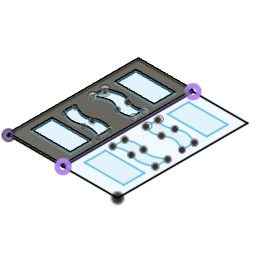
flaps final v2 (Autodesk Fusion 360 design; units mm, degrees)
Autodesk Fusion 360 part; units mm, degrees
sketch "Sketch1" plane through (0, 0, 0) normal (0, 0, 1) x (1, 0, 0)
  line L0 (0, 500) -> (0, 0)
  line L1 (0, 0) -> (210, 0)
  line L2 (210, 0) -> (210, 500)
  line L3 (210, 500) -> (0, 500)
  line L4 (210, 0) -> (210, 500)
  line L5 (420, 500) -> (420, 0)
  line L6 (210, 500) -> (420, 500)
  line L7 (420, 0) -> (210, 0)
  point P0 (420, 0)
  dimension "d1" = 210
  dimension "d2" = 500
  constraint coincident L0.end L1.start
  constraint vertical L0
  constraint perpendicular L0 L1
  constraint perpendicular L1 L2
  constraint perpendicular L0 L3
  constraint symmetric L0.end L2 L5.end
  constraint symmetric L0.start L2 L5.start
  constraint symmetric L0.end L2 P0
  constraint symmetric L1.end L2 L4.start
  constraint symmetric L3.start L2 L4.end
  measures "d1" distance of L0 L2
  measures "d2" distance of L1 L3
sketch "Sketch2" plane through (0, 0, 0) normal (0, 0, 1) x (1, 0, 0)
  line L0 (33.711, 456.9389) -> (183.711, 456.9389)
  line L1 (183.711, 456.9389) -> (183.711, 376.9389)
  line L2 (183.711, 376.9389) -> (33.711, 376.9389)
  line L3 (33.711, 376.9389) -> (33.711, 456.9389)
  line L4 (210, 0) -> (210, 500)
  line L5 (236.289, 456.9389) -> (236.289, 376.9389)
  line L6 (236.289, 376.9389) -> (386.289, 376.9389)
  line L7 (386.289, 456.9389) -> (236.289, 456.9389)
  line L8 (386.289, 376.9389) -> (386.289, 456.9389)
  dimension "d5" = 80
  dimension "d6" = 150
  constraint horizontal L0
  constraint vertical L1
  constraint horizontal L2
  constraint vertical L3
  constraint symmetric L0.start L4 L7.start
  constraint symmetric L0.end L4 L5.start
  constraint symmetric L1.end L4 L5.end
  constraint symmetric L2.end L4 L6.end
  measures "d5" distance of L0 L2
  measures "d6" distance of L1 L3
sketch "Sketch3" plane through (0, 0, 0) normal (0, 0, 1) x (1, 0, 0)
  line L0 (32.2529, 55.6107) -> (182.2529, 55.6107)
  line L1 (182.2529, 55.6107) -> (182.2529, 135.6107)
  line L2 (182.2529, 135.6107) -> (32.2529, 135.6107)
  line L3 (32.2529, 135.6107) -> (32.2529, 55.6107)
  line L4 (210, 0) -> (210, 500)
  line L5 (237.7471, 55.6107) -> (237.7471, 135.6107)
  line L6 (387.7471, 135.6107) -> (387.7471, 55.6107)
  line L7 (237.7471, 135.6107) -> (387.7471, 135.6107)
  line L8 (387.7471, 55.6107) -> (237.7471, 55.6107)
  dimension "d3" = 80
  dimension "d4" = 150
  constraint horizontal L0
  constraint vertical L1
  constraint horizontal L2
  constraint vertical L3
  constraint symmetric L0.start L4 L6.end
  constraint symmetric L0.end L4 L5.start
  constraint symmetric L1.end L4 L5.end
  constraint symmetric L2.end L4 L6.start
  measures "d3" distance of L0.end L1.end
  measures "d4" distance of L1 L3
sketch "Sketch4" plane through (0, 0, 0) normal (0, 0, 1) x (1, 0, 0)
  spline S0 degree 5 poles (37.1063, 332.6897) (42.3749, 335.3073) (52.3549, 339.9904) (65.6542, 345.3585) (80.2569, 349.3524) (94.455, 349.9181) (106.0588, 347.1834) (116.552, 342.4363) (127.2275, 337.0505) (138.9022, 332.4525) (151.9574, 330.0384) (163.6176, 330.8449) (173.049, 333.408) (179.6386, 336.0413) (183.0089, 337.5891) knots 0 0 0 0 0 0 0.1 0.2 0.3 0.4 0.5 0.6 0.7 0.8 0.9 1 1 1 1 1 1
  line L0 (12.8551, 320.6405) -> (61.3576, 344.7389)
  spline S1 degree 5 poles (37.1063, 285.0878) (42.8971, 288.4586) (53.8131, 294.4211) (68.19, 301.0281) (83.6155, 305.4358) (98.026, 305.1198) (109.2899, 300.9209) (119.1641, 294.9006) (129.1906, 289.0058) (140.3665, 284.7869) (153.15, 283.3608) (164.7942, 285.1007) (174.3242, 288.2578) (181.0276, 291.2129) (184.4668, 292.9031) knots 0 0 0 0 0 0 0.1 0.2 0.3 0.4 0.5 0.6 0.7 0.8 0.9 1 1 1 1 1 1
  line L1 (11.3971, 270.1228) -> (62.8155, 300.0529)
  line L2 (183.0089, 337.5891) -> (184.4668, 292.9031)
  line L3 (37.1063, 332.6897) -> (37.1063, 285.0878)
  spline S2 degree 5 poles (33.001, 177.9329) (38.3874, 175.2566) (48.5839, 170.5407) (62.1501, 165.3764) (77.0074, 162.0547) (91.4293, 162.4372) (103.2499, 165.5685) (114.0265, 169.6123) (125.0886, 172.9374) (137.2166, 174.4629) (150.704, 173.6089) (162.6105, 170.7864) (172.1303, 167.4148) (178.7303, 164.6061) (182.0937, 163.0615) knots 0 0 0 0 0 0 0.1 0.2 0.3 0.4 0.5 0.6 0.7 0.8 0.9 1 1 1 1 1 1
  line L4 (165.4289, 329.5156) -> (200.5889, 345.6626)
  line L5 (8.7497, 189.9821) -> (57.2522, 165.8837)
  line L6 (164.5136, 171.135) -> (199.6737, 154.988)
  line L7 (33.001, 177.9329) -> (33.001, 225.5347)
  spline S3 degree 5 poles (33.001, 225.5347) (38.5243, 222.3196) (48.8936, 216.5629) (62.4155, 209.9478) (76.6735, 204.9492) (89.8078, 203.8525) (100.2443, 206.3287) (109.9563, 210.6694) (120.5592, 215.2082) (132.869, 218.4944) (147.0982, 219.3055) (159.9368, 217.1832) (170.2893, 213.7191) (177.4957, 210.5385) (181.175, 208.7303) knots 0 0 0 0 0 0 0.1 0.2 0.3 0.4 0.5 0.6 0.7 0.8 0.9 1 1 1 1 1 1
  line L8 (166.2067, 283.9293) -> (202.727, 301.8769)
  line L9 (7.2917, 240.4998) -> (58.7102, 210.5696)
  line L10 (162.9149, 217.7041) -> (199.4352, 199.7565)
  line L11 (182.0937, 163.0615) -> (181.175, 208.7303)
  line L12 (210, 0) -> (210, 500)
  spline S4 degree 5 poles (382.8937, 332.6897) (377.6251, 335.3073) (367.6451, 339.9904) (354.3458, 345.3585) (339.7431, 349.3524) (325.545, 349.9181) (313.9412, 347.1834) (303.448, 342.4363) (292.7725, 337.0505) (281.0978, 332.4525) (268.0426, 330.0384) (256.3824, 330.8449) (246.951, 333.408) (240.3614, 336.0413) (236.9911, 337.5891) knots 0 0 0 0 0 0 0.1 0.2 0.3 0.4 0.5 0.6 0.7 0.8 0.9 1 1 1 1 1 1
  line L13 (407.1449, 320.6405) -> (358.6424, 344.7389)
  line L14 (254.5711, 329.5156) -> (219.4111, 345.6626)
  line L15 (382.8937, 332.6897) -> (382.8937, 285.0878)
  line L16 (237.9063, 163.0615) -> (238.825, 208.7303)
  line L17 (236.9911, 337.5891) -> (235.5332, 292.9031)
  spline S5 degree 5 poles (386.999, 177.9329) (381.6126, 175.2566) (371.4161, 170.5407) (357.8499, 165.3764) (342.9926, 162.0547) (328.5707, 162.4372) (316.7501, 165.5685) (305.9735, 169.6123) (294.9114, 172.9374) (282.7834, 174.4629) (269.296, 173.6089) (257.3895, 170.7864) (247.8697, 167.4148) (241.2697, 164.6061) (237.9063, 163.0615) knots 0 0 0 0 0 0 0.1 0.2 0.3 0.4 0.5 0.6 0.7 0.8 0.9 1 1 1 1 1 1
  line L18 (411.2503, 189.9821) -> (362.7478, 165.8837)
  line L19 (255.4864, 171.135) -> (220.3263, 154.988)
  spline S6 degree 5 poles (386.999, 225.5347) (381.4757, 222.3196) (371.1064, 216.5629) (357.5845, 209.9478) (343.3265, 204.9492) (330.1922, 203.8525) (319.7557, 206.3287) (310.0437, 210.6694) (299.4408, 215.2082) (287.131, 218.4944) (272.9018, 219.3055) (260.0632, 217.1832) (249.7107, 213.7191) (242.5043, 210.5385) (238.825, 208.7303) knots 0 0 0 0 0 0 0.1 0.2 0.3 0.4 0.5 0.6 0.7 0.8 0.9 1 1 1 1 1 1
  line L20 (412.7083, 240.4998) -> (361.2898, 210.5696)
  line L21 (257.0851, 217.7041) -> (220.5648, 199.7565)
  spline S7 degree 5 poles (382.8937, 285.0878) (377.1029, 288.4586) (366.1869, 294.4211) (351.81, 301.0281) (336.3845, 305.4358) (321.974, 305.1198) (310.7101, 300.9209) (300.8359, 294.9006) (290.8094, 289.0058) (279.6335, 284.7869) (266.85, 283.3608) (255.2058, 285.1007) (245.6758, 288.2578) (238.9724, 291.2129) (235.5332, 292.9031) knots 0 0 0 0 0 0 0.1 0.2 0.3 0.4 0.5 0.6 0.7 0.8 0.9 1 1 1 1 1 1
  line L22 (408.6029, 270.1228) -> (357.1845, 300.0529)
  line L23 (253.7933, 283.9293) -> (217.273, 301.8769)
  line L24 (386.999, 177.9329) -> (386.999, 225.5347)
  point P0 (120.393, 340.4922)
  point P1 (123.6058, 292.4233)
  point P2 (117.8255, 170.5984)
  point P3 (112.0744, 211.5163)
  point P4 (307.9256, 211.5163)
  point P5 (299.607, 340.4922)
  point P6 (302.1745, 170.5984)
  point P7 (296.3942, 292.4233)
  constraint midpoint S0.start L0
  constraint midpoint S1.start L1
  constraint vertical L3
  constraint midpoint S0.end L4
  constraint midpoint S1.end L8
  constraint symmetric S0.start L12 S4.start
  constraint symmetric P0 L12 P5
  constraint symmetric S0.end L12 S4.end
  constraint symmetric L0.start L12 L13.start
  constraint symmetric L0.end L12 L13.end
  constraint symmetric L1.start L12 L22.start
  constraint symmetric L1.end L12 L22.end
  constraint symmetric S1.start L12 L15.end
  constraint symmetric S1.end L12 L17.end
  constraint symmetric P1 L12 P7
  constraint symmetric S2.start L12 S5.start
  constraint symmetric P2 L12 P6
  constraint symmetric S2.end L12 L16.start
  constraint symmetric L4.start L12 L14.start
  constraint symmetric L4.end L12 L14.end
  constraint symmetric L5.start L12 L18.start
  constraint symmetric L5.end L12 L18.end
  constraint symmetric L6.start L12 L19.start
  constraint symmetric L6.end L12 L19.end
  constraint symmetric L7.end L12 S6.start
  constraint symmetric P3 L12 P4
  constraint symmetric S3.end L12 L16.end
  constraint symmetric L8.start L12 L23.start
  constraint symmetric L8.end L12 L23.end
  constraint symmetric L9.start L12 L20.start
  constraint symmetric L9.end L12 L20.end
  constraint symmetric L10.start L12 L21.start
  constraint symmetric L10.end L12 L21.end
sketch "Sketch5" plane through (0, 0, 0) normal (0, 0, 1) x (1, 0, 0)
  line L0 (36.9414, 334.4826) -> (36.9414, 288.2338)
  constraint vertical L0
sketch "Sketch6" plane through (0, 0, 0) normal (0, 0, 1) x (1, 0, 0)
  line L0 (182.7332, 343.5551) -> (182.7332, 300.0101)
  line L1 (210, 0) -> (210, 500)
  line L2 (237.2668, 343.5551) -> (237.2668, 300.0101)
  constraint vertical L0
  constraint symmetric L0.start L1 L2.start
  constraint symmetric L0.end L1 L2.end
extrude "Extrude1" add sketch "Sketch1" along normal blind 8 contours L0 L1 L2 L3 L4
extrude "Extrude2" cut sketch "Sketch4" along normal blind 50 contours S2 L7 S3 L11
extrude "Extrude3" cut sketch "Sketch3" along normal blind 50 contours L0 L1 L2 L3
extrude "Extrude4" cut sketch "Sketch2" along normal blind 50 contours L0 L1 L2 L3
extrude "Extrude5" cut sketch "Sketch4" along normal blind 20 contours S0 S1 L2 L3
